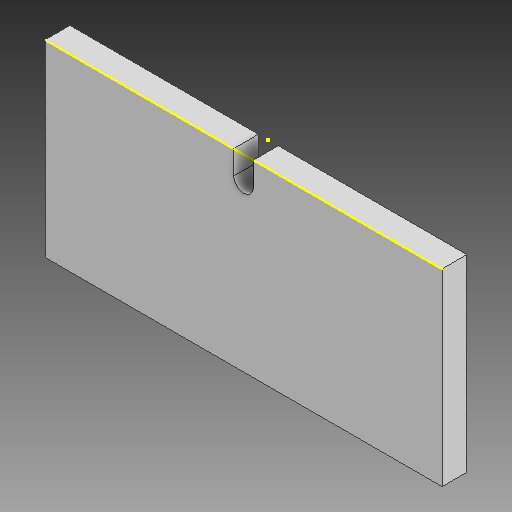
# Autodesk Inventor part: Verkleidungsdeckel
Saved by Autodesk Inventor 2021 (Build 250183000, 183)
## iProperties
Created: 2021-10-15
Part Number: Verkleidungsdeckel
Material: Generisch
Document SubType Name: Modeling
Designer: lukas
Density: 1 g/cm^3
Appearance: Vorgabe
Stock Number: Verkleidungsdeckel
Author: lukas
Autodesk Inventor part; units mm, degrees
ref_plane "YZ Plane" through (0, 0, 0) normal (1, 0, 0) x (0, 1, 0)
ref_plane "XZ Plane" through (0, 0, 0) normal (0, 1, 0) x (-1, 0, 0)
ref_plane "XY Plane" through (0, 0, 0) normal (0, 0, 1) x (1, 0, 0)
sketch "Skizze1" plane through (0, 0, 0) normal (0, 0, 1) x (1, 0, 0)
  line L0 (-280, 0) -> (280, 0) projected
  line L1 (0, -126.7237) -> (0, 179.8763) projected
  line L2 (-200, 107.0763) -> (200, 107.0763)
  line L3 (200, 107.0763) -> (200, -82.9237)
  line L4 (200, -82.9237) -> (-200, -82.9237)
  line L5 (-200, -82.9237) -> (-200, 107.0763)
  point P0 (0, 0)
  dimension "d0" = 190
  dimension "d1" = 400
  constraints: 8 end point, 2 parallel, 1 horizontal, 1 perpendicular, 1 other
  measures "d0" distance of L4.end L2.start
  measures "d1" distance of L3.end L4.end
extrude "Extrusion1" add sketch "Skizze1" along normal blind 25
sketch "Skizze2" plane through (-200, 107.0763, 0) normal (0, 1, 0) x (1, 0, 0)
  line L0 (0, -25) -> (400, -25) projected
  point P0 (200, 0)
sketch "Skizze4" plane through (0, 0, 0) normal (0, 0, -1) x (-1, 0, 0)
  line L0 (-200, 107.0763) -> (200, 107.0763) projected
  line L1 (-10, 107.0763) -> (10, 107.0763)
  line L2 (10, 107.0763) -> (10, 83.161)
  line L3 (10, 83.161) -> (-10, 83.161)
  line L4 (-10, 83.161) -> (-10, 107.0763)
  circle A0 centre (0, 83.161) radius 10
  point P0 (0, 0)
  dimension "d12" = 20
  dimension "d13" = 10
  constraints: 8 end point, 2 parallel, 1 horizontal, 1 midpoint, 1 perpendicular, 1 point on line, 3 other
  measures "d12" distance of L2.end L3.end
  measures "d13" distance from line of point (0, 0) L4
extrude "Extrusion3" cut sketch "Skizze4" against normal blind 25
